Autodesk Fusion 360 part; units mm, degrees
(part 3 of 3)
sketch "Sketch2 (22)" plane through (0, 0, 0) normal (0, 0, 1) x (1, 0, 0) in component "04_RobotArm (2)"
  line L0 (-45, 50, 120) -> (11, 50, 120)
  line L1 (11, 50, 120) -> (11, 106, 120)
  line L2 (11, 106, 120) -> (-45, 106, 120)
  line L3 (-45, 106, 120) -> (-45, 50, 120)
extrude "Extrude2'''''''''''''''''''''" add sketch "Sketch2 (22)" along normal blind 76 separate body contours L0 L1 L2 L3 in plane through (0, 0, 120) normal (0, 0, 1) makes body 220 in component "04_RobotArm (2)"
sketch "Sketch3 (20)" plane through (0, 0, 0) normal (0, 0, 1) x (1, 0, 0) in component "04_RobotArm (2)"
  line L0 (-20, -20, 190) -> (20, -20, 190)
  line L1 (20, -20, 190) -> (20, 20, 190)
  line L2 (20, 20, 190) -> (-20, 20, 190)
  line L3 (-20, 20, 190) -> (-20, -20, 190)
extrude "Extrude3'''''''''''''''''''" add sketch "Sketch3 (20)" along normal blind 400 separate body contours L0 L1 L2 L3 in plane through (0, 0, 190) normal (0, 0, 1) makes body 221 in component "04_RobotArm (2)"
sketch "Sketch4 (20)" plane through (0, 0, 0) normal (0, 0, 1) x (1, 0, 0) in component "04_RobotArm (2)"
  line L0 (-25, -25, 250) -> (25, -25, 250)
  line L1 (25, -25, 250) -> (25, 25, 250)
  line L2 (25, 25, 250) -> (-25, 25, 250)
  line L3 (-25, 25, 250) -> (-25, -25, 250)
extrude "Extrude4'''''''''''''''''''" add sketch "Sketch4 (20)" along normal blind 5 separate body contours L0 L1 L2 L3 in plane through (0, 0, 250) normal (0, 0, 1) makes body 222 in component "04_RobotArm (2)"
sketch "Sketch5 (17)" plane through (0, 0, 0) normal (0, 0, 1) x (1, 0, 0) in component "04_RobotArm (2)"
  line L0 (-25, -25, 350) -> (25, -25, 350)
  line L1 (25, -25, 350) -> (25, 25, 350)
  line L2 (25, 25, 350) -> (-25, 25, 350)
  line L3 (-25, 25, 350) -> (-25, -25, 350)
extrude "Extrude5''''''''''''''''" add sketch "Sketch5 (17)" along normal blind 5 separate body contours L0 L1 L2 L3 in plane through (0, 0, 350) normal (0, 0, 1) makes body 223 in component "04_RobotArm (2)"
sketch "Sketch6 (17)" plane through (0, 0, 0) normal (0, 0, 1) x (1, 0, 0) in component "04_RobotArm (2)"
  line L0 (-25, -25, 450) -> (25, -25, 450)
  line L1 (25, -25, 450) -> (25, 25, 450)
  line L2 (25, 25, 450) -> (-25, 25, 450)
  line L3 (-25, 25, 450) -> (-25, -25, 450)
extrude "Extrude6''''''''''''''''" add sketch "Sketch6 (17)" along normal blind 5 separate body contours L0 L1 L2 L3 in plane through (0, 0, 450) normal (0, 0, 1) makes body 224 in component "04_RobotArm (2)"
sketch "Sketch7 (17)" plane through (0, 0, 0) normal (0, 0, 1) x (1, 0, 0) in component "04_RobotArm (2)"
  circle A0 through (60, 0, 590) (-30, 51.9615, 590) (-30, -51.9615, 590)
extrude "Extrude7''''''''''''''''" add sketch "Sketch7 (17)" along normal blind 40 separate body contours A0 in plane through (0, 0, 590) normal (0, 0, 1) makes body 225 in component "04_RobotArm (2)"
sketch "Sketch8 (17)" plane through (0, 0, 0) normal (0, 0, 1) x (1, 0, 0) in component "04_RobotArm (2)"
  line L0 (50, -30, 570) -> (106, -30, 570)
  line L1 (106, -30, 570) -> (106, 26, 570)
  line L2 (106, 26, 570) -> (50, 26, 570)
  line L3 (50, 26, 570) -> (50, -30, 570)
extrude "Extrude8''''''''''''''''" add sketch "Sketch8 (17)" along normal blind 76 separate body contours L0 L1 L2 L3 in plane through (0, 0, 570) normal (0, 0, 1) makes body 226 in component "04_RobotArm (2)"
sketch "Sketch9 (17)" plane through (0, 0, 0) normal (0, 0, 1) x (1, 0, 0) in component "04_RobotArm (2)"
  line L0 (-20, -20, 630) -> (20, -20, 630)
  line L1 (20, -20, 630) -> (20, 20, 630)
  line L2 (20, 20, 630) -> (-20, 20, 630)
  line L3 (-20, 20, 630) -> (-20, -20, 630)
extrude "Extrude9''''''''''''''''" add sketch "Sketch9 (17)" along normal blind 350 separate body contours L0 L1 L2 L3 in plane through (0, 0, 630) normal (0, 0, 1) makes body 227 in component "04_RobotArm (2)"
sketch "Sketch10 (17)" plane through (0, 0, 0) normal (0, 0, 1) x (1, 0, 0) in component "04_RobotArm (2)"
  circle A0 through (50, 0, 980) (-25, 43.3013, 980) (-25, -43.3013, 980)
extrude "Extrude10''''''''''''''''" add sketch "Sketch10 (17)" along normal blind 30 separate body contours A0 in plane through (0, 0, 980) normal (0, 0, 1) makes body 228 in component "04_RobotArm (2)"
sketch "Sketch11 (9)" plane through (0, 0, 0) normal (0, 0, 1) x (1, 0, 0) in component "04_RobotArm (2)"
  line L0 (30, -20, 960) -> (70, -20, 960)
  line L1 (70, -20, 960) -> (70, 20, 960)
  line L2 (70, 20, 960) -> (30, 20, 960)
  line L3 (30, 20, 960) -> (30, -20, 960)
extrude "Extrude11''''''''" add sketch "Sketch11 (9)" along normal blind 50 separate body contours L0 L1 L2 L3 in plane through (0, 0, 960) normal (0, 0, 1) makes body 229 in component "04_RobotArm (2)"
sketch "Sketch12 (7)" plane through (0, 0, 0) normal (0, 0, 1) x (1, 0, 0) in component "04_RobotArm (2)"
  circle A0 through (-15, 30, 130) (-37.5, 42.9904, 130) (-37.5, 17.0096, 130)
extrude "Extrude12''''''" add sketch "Sketch12 (7)" along normal blind 15 separate body contours A0 in plane through (0, 0, 130) normal (0, 0, 1) makes body 230 in component "04_RobotArm (2)"
sketch "Sketch13 (7)" plane through (0, 0, 0) normal (0, 0, 1) x (1, 0, 0) in component "04_RobotArm (2)"
  circle A0 through (-15, 30, 570) (-37.5, 42.9904, 570) (-37.5, 17.0096, 570)
extrude "Extrude13''''''" add sketch "Sketch13 (7)" along normal blind 15 separate body contours A0 in plane through (0, 0, 570) normal (0, 0, 1) makes body 231 in component "04_RobotArm (2)"
sketch "Sketch14 (7)" plane through (0, 0, 0) normal (0, 0, 1) x (1, 0, 0) in component "04_RobotArm (2)"
  circle A0 through (-15, 30, 960) (-37.5, 42.9904, 960) (-37.5, 17.0096, 960)
extrude "Extrude14''''''" add sketch "Sketch14 (7)" along normal blind 15 separate body contours A0 in plane through (0, 0, 960) normal (0, 0, 1) makes body 232 in component "04_RobotArm (2)"
sketch "Sketch1 (23)" plane through (0, 0, 0) normal (0, 0, 1) x (1, 0, 0) in component "05_Gripper (2)"
  line L0 (-50, -30) -> (50, -30)
  line L1 (50, -30) -> (50, 30)
  line L2 (50, 30) -> (-50, 30)
  line L3 (-50, 30) -> (-50, -30)
extrude "Extrude1''''''''''''''''''''''" add sketch "Sketch1 (23)" along normal blind 60 separate body makes body 233 in component "05_Gripper (2)"
sketch "Sketch2 (23)" plane through (0, 0, 0) normal (0, 0, 1) x (1, 0, 0) in component "05_Gripper (2)"
  line L0 (-75, -30) -> (-50, -30)
  line L1 (-50, -30) -> (-50, 30)
  line L2 (-50, 30) -> (-75, 30)
  line L3 (-75, 30) -> (-75, -30)
extrude "Extrude2''''''''''''''''''''''" add sketch "Sketch2 (23)" along normal blind 50 separate body makes body 234 in component "05_Gripper (2)"
sketch "Sketch3 (21)" plane through (0, 0, 0) normal (0, 0, 1) x (1, 0, 0) in component "05_Gripper (2)"
  line L0 (50, -30) -> (75, -30)
  line L1 (75, -30) -> (75, 30)
  line L2 (75, 30) -> (50, 30)
  line L3 (50, 30) -> (50, -30)
extrude "Extrude3''''''''''''''''''''" add sketch "Sketch3 (21)" along normal blind 50 separate body makes body 235 in component "05_Gripper (2)"
sketch "Sketch4 (21)" plane through (0, 0, 0) normal (0, 0, 1) x (1, 0, 0) in component "05_Gripper (2)"
  line L0 (-50, -25, 10) -> (50, -25, 10)
  line L1 (50, -25, 10) -> (50, -21, 10)
  line L2 (50, -21, 10) -> (-50, -21, 10)
  line L3 (-50, -21, 10) -> (-50, -25, 10)
extrude "Extrude4''''''''''''''''''''" add sketch "Sketch4 (21)" along normal blind 30 separate body contours L0 L1 L2 L3 in plane through (0, 0, 10) normal (0, 0, 1) makes body 236 in component "05_Gripper (2)"
sketch "Sketch5 (18)" plane through (0, 0, 0) normal (0, 0, 1) x (1, 0, 0) in component "05_Gripper (2)"
  line L0 (-50, 25, 10) -> (50, 25, 10)
  line L1 (50, 25, 10) -> (50, 29, 10)
  line L2 (50, 29, 10) -> (-50, 29, 10)
  line L3 (-50, 29, 10) -> (-50, 25, 10)
extrude "Extrude5'''''''''''''''''" add sketch "Sketch5 (18)" along normal blind 30 separate body contours L0 L1 L2 L3 in plane through (0, 0, 10) normal (0, 0, 1) makes body 237 in component "05_Gripper (2)"
sketch "Sketch6 (18)" plane through (0, 0, 0) normal (0, 0, 1) x (1, 0, 0) in component "05_Gripper (2)"
  circle A0 through (25, 0, 60) (-12.5, 21.6506, 60) (-12.5, -21.6506, 60)
extrude "Extrude6'''''''''''''''''" add sketch "Sketch6 (18)" along normal blind 80 separate body contours A0 in plane through (0, 0, 60) normal (0, 0, 1) makes body 238 in component "05_Gripper (2)"
sketch "Sketch7 (18)" plane through (0, 0, 0) normal (0, 0, 1) x (1, 0, 0) in component "05_Gripper (2)"
  circle A0 through (-16, 0, 140) (-22, 3.4641, 140) (-22, -3.4641, 140)
extrude "Extrude7'''''''''''''''''" add sketch "Sketch7 (18)" along normal blind 30 separate body contours A0 in plane through (0, 0, 140) normal (0, 0, 1) makes body 239 in component "05_Gripper (2)"
sketch "Sketch8 (18)" plane through (0, 0, 0) normal (0, 0, 1) x (1, 0, 0) in component "05_Gripper (2)"
  circle A0 through (24, 0, 140) (18, 3.4641, 140) (18, -3.4641, 140)
extrude "Extrude8'''''''''''''''''" add sketch "Sketch8 (18)" along normal blind 30 separate body contours A0 in plane through (0, 0, 140) normal (0, 0, 1) makes body 240 in component "05_Gripper (2)"
sketch "Sketch9 (18)" plane through (0, 0, 0) normal (0, 0, 1) x (1, 0, 0) in component "05_Gripper (2)"
  circle A0 through (30, 0, -20) (-15, 25.9808, -20) (-15, -25.9808, -20)
extrude "Extrude9'''''''''''''''''" add sketch "Sketch9 (18)" along normal blind 20 separate body contours A0 in plane through (0, 0, -20) normal (0, 0, 1) makes body 241 in component "05_Gripper (2)"
sketch "Sketch10 (18)" plane through (0, 0, 0) normal (0, 0, 1) x (1, 0, 0) in component "05_Gripper (2)"
  line L0 (-10, -5, -5) -> (10, -5, -5)
  line L1 (10, -5, -5) -> (10, 5, -5)
  line L2 (10, 5, -5) -> (-10, 5, -5)
  line L3 (-10, 5, -5) -> (-10, -5, -5)
extrude "Extrude10'''''''''''''''''" add sketch "Sketch10 (18)" along normal blind 3 separate body contours L0 L1 L2 L3 in plane through (0, 0, -5) normal (0, 0, 1) makes body 242 in component "05_Gripper (2)"
sketch "Sketch11 (10)" plane through (0, 0, 0) normal (0, 0, 1) x (1, 0, 0) in component "05_Gripper (2)"
  line L0 (-35, 35, 20) -> (35, 35, 20)
  line L1 (35, 35, 20) -> (35, 65, 20)
  line L2 (35, 65, 20) -> (-35, 65, 20)
  line L3 (-35, 65, 20) -> (-35, 35, 20)
extrude "Extrude11'''''''''" add sketch "Sketch11 (10)" along normal blind 40 separate body contours L0 L1 L2 L3 in plane through (0, 0, 20) normal (0, 0, 1) makes body 243 in component "05_Gripper (2)"
sketch "Sketch1 (24)" plane through (0, 0, 0) normal (0, 0, 1) x (1, 0, 0) in component "06_SortingBins (2)"
  line L0 (396.8309, 88.1111) -> (636.8309, 88.1111)
  line L1 (636.8309, 88.1111) -> (636.8309, 288.1111)
  line L2 (636.8309, 288.1111) -> (396.8309, 288.1111)
  line L3 (396.8309, 288.1111) -> (396.8309, 88.1111)
extrude "Extrude1'''''''''''''''''''''''" add sketch "Sketch1 (24)" along normal blind 250 separate body makes body 244 in component "06_SortingBins (2)"
sketch "Sketch2 (24)" plane through (0, 0, 0) normal (0, 0, 1) x (1, 0, 0) in component "06_SortingBins (2)"
  line L0 (456.8309, 83.1111, 80) -> (576.8309, 83.1111, 80)
  line L1 (576.8309, 83.1111, 80) -> (576.8309, 86.1111, 80)
  line L2 (576.8309, 86.1111, 80) -> (456.8309, 86.1111, 80)
  line L3 (456.8309, 86.1111, 80) -> (456.8309, 83.1111, 80)
extrude "Extrude2'''''''''''''''''''''''" add sketch "Sketch2 (24)" along normal blind 60 separate body contours L0 L1 L2 L3 in plane through (0, 0, 80) normal (0, 0, 1) makes body 245 in component "06_SortingBins (2)"
sketch "Sketch3 (22)" plane through (0, 0, 0) normal (0, 0, 1) x (1, 0, 0) in component "06_SortingBins (2)"
  line L0 (396.8309, 88.1111, -15) -> (636.8309, 88.1111, -15)
  line L1 (636.8309, 88.1111, -15) -> (636.8309, 288.1111, -15)
  line L2 (636.8309, 288.1111, -15) -> (396.8309, 288.1111, -15)
  line L3 (396.8309, 288.1111, -15) -> (396.8309, 88.1111, -15)
extrude "Extrude3'''''''''''''''''''''" add sketch "Sketch3 (22)" along normal blind 15 separate body contours L0 L1 L2 L3 in plane through (0, 0, -15) normal (0, 0, 1) makes body 246 in component "06_SortingBins (2)"
sketch "Sketch4 (22)" plane through (0, 0, 0) normal (0, 0, 1) x (1, 0, 0) in component "06_SortingBins (2)"
  line L0 (280.0555, 277.4329) -> (520.0555, 277.4329)
  line L1 (520.0555, 277.4329) -> (520.0555, 477.4329)
  line L2 (520.0555, 477.4329) -> (280.0555, 477.4329)
  line L3 (280.0555, 477.4329) -> (280.0555, 277.4329)
extrude "Extrude4'''''''''''''''''''''" add sketch "Sketch4 (22)" along normal blind 250 separate body makes body 247 in component "06_SortingBins (2)"
sketch "Sketch5 (19)" plane through (0, 0, 0) normal (0, 0, 1) x (1, 0, 0) in component "06_SortingBins (2)"
  line L0 (340.0555, 272.4329, 80) -> (460.0555, 272.4329, 80)
  line L1 (460.0555, 272.4329, 80) -> (460.0555, 275.4329, 80)
  line L2 (460.0555, 275.4329, 80) -> (340.0555, 275.4329, 80)
  line L3 (340.0555, 275.4329, 80) -> (340.0555, 272.4329, 80)
extrude "Extrude5''''''''''''''''''" add sketch "Sketch5 (19)" along normal blind 60 separate body contours L0 L1 L2 L3 in plane through (0, 0, 80) normal (0, 0, 1) makes body 248 in component "06_SortingBins (2)"
sketch "Sketch6 (19)" plane through (0, 0, 0) normal (0, 0, 1) x (1, 0, 0) in component "06_SortingBins (2)"
  line L0 (280.0555, 277.4329, -15) -> (520.0555, 277.4329, -15)
  line L1 (520.0555, 277.4329, -15) -> (520.0555, 477.4329, -15)
  line L2 (520.0555, 477.4329, -15) -> (280.0555, 477.4329, -15)
  line L3 (280.0555, 477.4329, -15) -> (280.0555, 277.4329, -15)
extrude "Extrude6''''''''''''''''''" add sketch "Sketch6 (19)" along normal blind 15 separate body contours L0 L1 L2 L3 in plane through (0, 0, -15) normal (0, 0, 1) makes body 249 in component "06_SortingBins (2)"
sketch "Sketch7 (19)" plane through (0, 0, 0) normal (0, 0, 1) x (1, 0, 0) in component "06_SortingBins (2)"
  line L0 (97.8439, 405.0189) -> (337.8439, 405.0189)
  line L1 (337.8439, 405.0189) -> (337.8439, 605.0189)
  line L2 (337.8439, 605.0189) -> (97.8439, 605.0189)
  line L3 (97.8439, 605.0189) -> (97.8439, 405.0189)
extrude "Extrude7''''''''''''''''''" add sketch "Sketch7 (19)" along normal blind 250 separate body makes body 250 in component "06_SortingBins (2)"
sketch "Sketch8 (19)" plane through (0, 0, 0) normal (0, 0, 1) x (1, 0, 0) in component "06_SortingBins (2)"
  line L0 (157.8439, 400.0189, 80) -> (277.8439, 400.0189, 80)
  line L1 (277.8439, 400.0189, 80) -> (277.8439, 403.0189, 80)
  line L2 (277.8439, 403.0189, 80) -> (157.8439, 403.0189, 80)
  line L3 (157.8439, 403.0189, 80) -> (157.8439, 400.0189, 80)
extrude "Extrude8''''''''''''''''''" add sketch "Sketch8 (19)" along normal blind 60 separate body contours L0 L1 L2 L3 in plane through (0, 0, 80) normal (0, 0, 1) makes body 251 in component "06_SortingBins (2)"
sketch "Sketch9 (19)" plane through (0, 0, 0) normal (0, 0, 1) x (1, 0, 0) in component "06_SortingBins (2)"
  line L0 (97.8439, 405.0189, -15) -> (337.8439, 405.0189, -15)
  line L1 (337.8439, 405.0189, -15) -> (337.8439, 605.0189, -15)
  line L2 (337.8439, 605.0189, -15) -> (97.8439, 605.0189, -15)
  line L3 (97.8439, 605.0189, -15) -> (97.8439, 405.0189, -15)
extrude "Extrude9''''''''''''''''''" add sketch "Sketch9 (19)" along normal blind 15 separate body contours L0 L1 L2 L3 in plane through (0, 0, -15) normal (0, 0, 1) makes body 252 in component "06_SortingBins (2)"
sketch "Sketch10 (19)" plane through (0, 0, 0) normal (0, 0, 1) x (1, 0, 0) in component "06_SortingBins (2)"
  line L0 (-120, 450) -> (120, 450)
  line L1 (120, 450) -> (120, 650)
  line L2 (120, 650) -> (-120, 650)
  line L3 (-120, 650) -> (-120, 450)
extrude "Extrude10''''''''''''''''''" add sketch "Sketch10 (19)" along normal blind 250 separate body makes body 253 in component "06_SortingBins (2)"
sketch "Sketch11 (11)" plane through (0, 0, 0) normal (0, 0, 1) x (1, 0, 0) in component "06_SortingBins (2)"
  line L0 (-60, 445, 80) -> (60, 445, 80)
  line L1 (60, 445, 80) -> (60, 448, 80)
  line L2 (60, 448, 80) -> (-60, 448, 80)
  line L3 (-60, 448, 80) -> (-60, 445, 80)
extrude "Extrude11''''''''''" add sketch "Sketch11 (11)" along normal blind 60 separate body contours L0 L1 L2 L3 in plane through (0, 0, 80) normal (0, 0, 1) makes body 254 in component "06_SortingBins (2)"
sketch "Sketch12 (8)" plane through (0, 0, 0) normal (0, 0, 1) x (1, 0, 0) in component "06_SortingBins (2)"
  line L0 (-120, 450, -15) -> (120, 450, -15)
  line L1 (120, 450, -15) -> (120, 650, -15)
  line L2 (120, 650, -15) -> (-120, 650, -15)
  line L3 (-120, 650, -15) -> (-120, 450, -15)
extrude "Extrude12'''''''" add sketch "Sketch12 (8)" along normal blind 15 separate body contours L0 L1 L2 L3 in plane through (0, 0, -15) normal (0, 0, 1) makes body 255 in component "06_SortingBins (2)"
sketch "Sketch13 (8)" plane through (0, 0, 0) normal (0, 0, 1) x (1, 0, 0) in component "06_SortingBins (2)"
  line L0 (-337.8439, 405.0189) -> (-97.8439, 405.0189)
  line L1 (-97.8439, 405.0189) -> (-97.8439, 605.0189)
  line L2 (-97.8439, 605.0189) -> (-337.8439, 605.0189)
  line L3 (-337.8439, 605.0189) -> (-337.8439, 405.0189)
extrude "Extrude13'''''''" add sketch "Sketch13 (8)" along normal blind 250 separate body makes body 256 in component "06_SortingBins (2)"
sketch "Sketch14 (8)" plane through (0, 0, 0) normal (0, 0, 1) x (1, 0, 0) in component "06_SortingBins (2)"
  line L0 (-277.8439, 400.0189, 80) -> (-157.8439, 400.0189, 80)
  line L1 (-157.8439, 400.0189, 80) -> (-157.8439, 403.0189, 80)
  line L2 (-157.8439, 403.0189, 80) -> (-277.8439, 403.0189, 80)
  line L3 (-277.8439, 403.0189, 80) -> (-277.8439, 400.0189, 80)
extrude "Extrude14'''''''" add sketch "Sketch14 (8)" along normal blind 60 separate body contours L0 L1 L2 L3 in plane through (0, 0, 80) normal (0, 0, 1) makes body 257 in component "06_SortingBins (2)"
sketch "Sketch15 (5)" plane through (0, 0, 0) normal (0, 0, 1) x (1, 0, 0) in component "06_SortingBins (2)"
  line L0 (-337.8439, 405.0189, -15) -> (-97.8439, 405.0189, -15)
  line L1 (-97.8439, 405.0189, -15) -> (-97.8439, 605.0189, -15)
  line L2 (-97.8439, 605.0189, -15) -> (-337.8439, 605.0189, -15)
  line L3 (-337.8439, 605.0189, -15) -> (-337.8439, 405.0189, -15)
extrude "Extrude15''''" add sketch "Sketch15 (5)" along normal blind 15 separate body contours L0 L1 L2 L3 in plane through (0, 0, -15) normal (0, 0, 1) makes body 258 in component "06_SortingBins (2)"
sketch "Sketch16 (3)" plane through (0, 0, 0) normal (0, 0, 1) x (1, 0, 0) in component "06_SortingBins (2)"
  line L0 (-520.0555, 277.4329) -> (-280.0555, 277.4329)
  line L1 (-280.0555, 277.4329) -> (-280.0555, 477.4329)
  line L2 (-280.0555, 477.4329) -> (-520.0555, 477.4329)
  line L3 (-520.0555, 477.4329) -> (-520.0555, 277.4329)
extrude "Extrude16''" add sketch "Sketch16 (3)" along normal blind 250 separate body makes body 259 in component "06_SortingBins (2)"
sketch "Sketch17 (3)" plane through (0, 0, 0) normal (0, 0, 1) x (1, 0, 0) in component "06_SortingBins (2)"
  line L0 (-460.0555, 272.4329, 80) -> (-340.0555, 272.4329, 80)
  line L1 (-340.0555, 272.4329, 80) -> (-340.0555, 275.4329, 80)
  line L2 (-340.0555, 275.4329, 80) -> (-460.0555, 275.4329, 80)
  line L3 (-460.0555, 275.4329, 80) -> (-460.0555, 272.4329, 80)
extrude "Extrude17''" add sketch "Sketch17 (3)" along normal blind 60 separate body contours L0 L1 L2 L3 in plane through (0, 0, 80) normal (0, 0, 1) makes body 260 in component "06_SortingBins (2)"
sketch "Sketch18 (3)" plane through (0, 0, 0) normal (0, 0, 1) x (1, 0, 0) in component "06_SortingBins (2)"
  line L0 (-520.0555, 277.4329, -15) -> (-280.0555, 277.4329, -15)
  line L1 (-280.0555, 277.4329, -15) -> (-280.0555, 477.4329, -15)
  line L2 (-280.0555, 477.4329, -15) -> (-520.0555, 477.4329, -15)
  line L3 (-520.0555, 477.4329, -15) -> (-520.0555, 277.4329, -15)
extrude "Extrude18''" add sketch "Sketch18 (3)" along normal blind 15 separate body contours L0 L1 L2 L3 in plane through (0, 0, -15) normal (0, 0, 1) makes body 261 in component "06_SortingBins (2)"
sketch "Sketch19 (3)" plane through (0, 0, 0) normal (0, 0, 1) x (1, 0, 0) in component "06_SortingBins (2)"
  line L0 (-636.8309, 88.1111) -> (-396.8309, 88.1111)
  line L1 (-396.8309, 88.1111) -> (-396.8309, 288.1111)
  line L2 (-396.8309, 288.1111) -> (-636.8309, 288.1111)
  line L3 (-636.8309, 288.1111) -> (-636.8309, 88.1111)
extrude "Extrude19''" add sketch "Sketch19 (3)" along normal blind 250 separate body makes body 262 in component "06_SortingBins (2)"
sketch "Sketch20 (3)" plane through (0, 0, 0) normal (0, 0, 1) x (1, 0, 0) in component "06_SortingBins (2)"
  line L0 (-576.8309, 83.1111, 80) -> (-456.8309, 83.1111, 80)
  line L1 (-456.8309, 83.1111, 80) -> (-456.8309, 86.1111, 80)
  line L2 (-456.8309, 86.1111, 80) -> (-576.8309, 86.1111, 80)
  line L3 (-576.8309, 86.1111, 80) -> (-576.8309, 83.1111, 80)
extrude "Extrude20''" add sketch "Sketch20 (3)" along normal blind 60 separate body contours L0 L1 L2 L3 in plane through (0, 0, 80) normal (0, 0, 1) makes body 263 in component "06_SortingBins (2)"
sketch "Sketch21 (3)" plane through (0, 0, 0) normal (0, 0, 1) x (1, 0, 0) in component "06_SortingBins (2)"
  line L0 (-636.8309, 88.1111, -15) -> (-396.8309, 88.1111, -15)
  line L1 (-396.8309, 88.1111, -15) -> (-396.8309, 288.1111, -15)
  line L2 (-396.8309, 288.1111, -15) -> (-636.8309, 288.1111, -15)
  line L3 (-636.8309, 288.1111, -15) -> (-636.8309, 88.1111, -15)
extrude "Extrude21''" add sketch "Sketch21 (3)" along normal blind 15 separate body contours L0 L1 L2 L3 in plane through (0, 0, -15) normal (0, 0, 1) makes body 264 in component "06_SortingBins (2)"
sketch "Sketch1 (25)" plane through (0, 0, 0) normal (0, 0, 1) x (1, 0, 0) in component "07_ComputeCabinet (2)"
  line L0 (0, 0) -> (500, 0)
  line L1 (500, 0) -> (500, 300)
  line L2 (500, 300) -> (0, 300)
  line L3 (0, 300) -> (0, 0)
extrude "Extrude1''''''''''''''''''''''''" add sketch "Sketch1 (25)" along normal blind 700 separate body makes body 265 in component "07_ComputeCabinet (2)"
sketch "Sketch2 (25)" plane through (0, 0, 0) normal (0, 0, 1) x (1, 0, 0) in component "07_ComputeCabinet (2)"
  line L0 (0, -5, 50) -> (500, -5, 50)
  line L1 (500, -5, 50) -> (500, 0, 50)
  line L2 (500, 0, 50) -> (0, 0, 50)
  line L3 (0, 0, 50) -> (0, -5, 50)
extrude "Extrude2''''''''''''''''''''''''" add sketch "Sketch2 (25)" along normal blind 600 separate body contours L0 L1 L2 L3 in plane through (0, 0, 50) normal (0, 0, 1) makes body 266 in component "07_ComputeCabinet (2)"
sketch "Sketch3 (23)" plane through (0, 0, 0) normal (0, 0, 1) x (1, 0, 0) in component "07_ComputeCabinet (2)"
  line L0 (30, 50, 120) -> (470, 50, 120)
  line L1 (470, 50, 120) -> (470, 54, 120)
  line L2 (470, 54, 120) -> (30, 54, 120)
  line L3 (30, 54, 120) -> (30, 50, 120)
extrude "Extrude3''''''''''''''''''''''" add sketch "Sketch3 (23)" along normal blind 15 separate body contours L0 L1 L2 L3 in plane through (0, 0, 120) normal (0, 0, 1) makes body 267 in component "07_ComputeCabinet (2)"
sketch "Sketch4 (23)" plane through (0, 0, 0) normal (0, 0, 1) x (1, 0, 0) in component "07_ComputeCabinet (2)"
  line L0 (30, 50, 300) -> (470, 50, 300)
  line L1 (470, 50, 300) -> (470, 54, 300)
  line L2 (470, 54, 300) -> (30, 54, 300)
  line L3 (30, 54, 300) -> (30, 50, 300)
extrude "Extrude4''''''''''''''''''''''" add sketch "Sketch4 (23)" along normal blind 15 separate body contours L0 L1 L2 L3 in plane through (0, 0, 300) normal (0, 0, 1) makes body 268 in component "07_ComputeCabinet (2)"
sketch "Sketch5 (20)" plane through (0, 0, 0) normal (0, 0, 1) x (1, 0, 0) in component "07_ComputeCabinet (2)"
  line L0 (30, 50, 500) -> (470, 50, 500)
  line L1 (470, 50, 500) -> (470, 54, 500)
  line L2 (470, 54, 500) -> (30, 54, 500)
  line L3 (30, 54, 500) -> (30, 50, 500)
extrude "Extrude5'''''''''''''''''''" add sketch "Sketch5 (20)" along normal blind 15 separate body contours L0 L1 L2 L3 in plane through (0, 0, 500) normal (0, 0, 1) makes body 269 in component "07_ComputeCabinet (2)"
sketch "Sketch6 (20)" plane through (0, 0, 0) normal (0, 0, 1) x (1, 0, 0) in component "07_ComputeCabinet (2)"
  line L0 (40, 60, 140) -> (140, 60, 140)
  line L1 (140, 60, 140) -> (140, 140, 140)
  line L2 (140, 140, 140) -> (40, 140, 140)
  line L3 (40, 140, 140) -> (40, 60, 140)
extrude "Extrude6'''''''''''''''''''" add sketch "Sketch6 (20)" along normal blind 60 separate body contours L0 L1 L2 L3 in plane through (0, 0, 140) normal (0, 0, 1) makes body 270 in component "07_ComputeCabinet (2)"
sketch "Sketch7 (20)" plane through (0, 0, 0) normal (0, 0, 1) x (1, 0, 0) in component "07_ComputeCabinet (2)"
  circle A0 through (120, 100, 200) (75, 125.9808, 200) (75, 74.0192, 200)
extrude "Extrude7'''''''''''''''''''" add sketch "Sketch7 (20)" along normal blind 10 separate body contours A0 in plane through (0, 0, 200) normal (0, 0, 1) makes body 271 in component "07_ComputeCabinet (2)"
sketch "Sketch8 (20)" plane through (0, 0, 0) normal (0, 0, 1) x (1, 0, 0) in component "07_ComputeCabinet (2)"
  line L0 (180, 60, 140) -> (240, 60, 140)
  line L1 (240, 60, 140) -> (240, 100, 140)
  line L2 (240, 100, 140) -> (180, 100, 140)
  line L3 (180, 100, 140) -> (180, 60, 140)
extrude "Extrude8'''''''''''''''''''" add sketch "Sketch8 (20)" along normal blind 10 separate body contours L0 L1 L2 L3 in plane through (0, 0, 140) normal (0, 0, 1) makes body 272 in component "07_ComputeCabinet (2)"
sketch "Sketch9 (20)" plane through (0, 0, 0) normal (0, 0, 1) x (1, 0, 0) in component "07_ComputeCabinet (2)"
  line L0 (270, 60, 140) -> (350, 60, 140)
  line L1 (350, 60, 140) -> (350, 80, 140)
  line L2 (350, 80, 140) -> (270, 80, 140)
  line L3 (270, 80, 140) -> (270, 60, 140)
extrude "Extrude9'''''''''''''''''''" add sketch "Sketch9 (20)" along normal blind 4 separate body contours L0 L1 L2 L3 in plane through (0, 0, 140) normal (0, 0, 1) makes body 273 in component "07_ComputeCabinet (2)"
sketch "Sketch10 (20)" plane through (0, 0, 0) normal (0, 0, 1) x (1, 0, 0) in component "07_ComputeCabinet (2)"
  line L0 (40, 60, 320) -> (220, 60, 320)
  line L1 (220, 60, 320) -> (220, 160, 320)
  line L2 (220, 160, 320) -> (40, 160, 320)
  line L3 (40, 160, 320) -> (40, 60, 320)
extrude "Extrude10'''''''''''''''''''" add sketch "Sketch10 (20)" along normal blind 60 separate body contours L0 L1 L2 L3 in plane through (0, 0, 320) normal (0, 0, 1) makes body 274 in component "07_ComputeCabinet (2)"
sketch "Sketch11 (12)" plane through (0, 0, 0) normal (0, 0, 1) x (1, 0, 0) in component "07_ComputeCabinet (2)"
  line L0 (260, 60, 320) -> (440, 60, 320)
  line L1 (440, 60, 320) -> (440, 160, 320)
  line L2 (440, 160, 320) -> (260, 160, 320)
  line L3 (260, 160, 320) -> (260, 60, 320)
extrude "Extrude11'''''''''''" add sketch "Sketch11 (12)" along normal blind 60 separate body contours L0 L1 L2 L3 in plane through (0, 0, 320) normal (0, 0, 1) makes body 275 in component "07_ComputeCabinet (2)"
sketch "Sketch12 (9)" plane through (0, 0, 0) normal (0, 0, 1) x (1, 0, 0) in component "07_ComputeCabinet (2)"
  line L0 (40, 60, 520) -> (420, 60, 520)
  line L1 (420, 60, 520) -> (420, 200, 520)
  line L2 (420, 200, 520) -> (40, 200, 520)
  line L3 (40, 200, 520) -> (40, 60, 520)
extrude "Extrude12''''''''" add sketch "Sketch12 (9)" along normal blind 100 separate body contours L0 L1 L2 L3 in plane through (0, 0, 520) normal (0, 0, 1) makes body 276 in component "07_ComputeCabinet (2)"
sketch "Sketch13 (9)" plane through (0, 0, 0) normal (0, 0, 1) x (1, 0, 0) in component "07_ComputeCabinet (2)"
  circle A0 through (80, -3, 550) (35, 22.9808, 550) (35, -28.9808, 550)
extrude "Extrude13''''''''" add sketch "Sketch13 (9)" along normal blind 30 separate body contours A0 in plane through (0, 0, 550) normal (0, 0, 1) makes body 277 in component "07_ComputeCabinet (2)"
sketch "Sketch14 (9)" plane through (0, 0, 0) normal (0, 0, 1) x (1, 0, 0) in component "07_ComputeCabinet (2)"
  line L0 (360, 60, 140) -> (420, 60, 140)
  line L1 (420, 60, 140) -> (420, 100, 140)
  line L2 (420, 100, 140) -> (360, 100, 140)
  line L3 (360, 100, 140) -> (360, 60, 140)
extrude "Extrude14''''''''" add sketch "Sketch14 (9)" along normal blind 40 separate body contours L0 L1 L2 L3 in plane through (0, 0, 140) normal (0, 0, 1) makes body 278 in component "07_ComputeCabinet (2)"
sketch "Sketch15 (6)" plane through (0, 0, 0) normal (0, 0, 1) x (1, 0, 0) in component "07_ComputeCabinet (2)"
  line L0 (180, 60, 220) -> (220, 60, 220)
  line L1 (220, 60, 220) -> (220, 85, 220)
  line L2 (220, 85, 220) -> (180, 85, 220)
  line L3 (180, 85, 220) -> (180, 60, 220)
extrude "Extrude15'''''" add sketch "Sketch15 (6)" along normal blind 3 separate body contours L0 L1 L2 L3 in plane through (0, 0, 220) normal (0, 0, 1) makes body 279 in component "07_ComputeCabinet (2)"
sketch "Sketch1 (26)" plane through (0, 0, 0) normal (0, 0, 1) x (1, 0, 0) in component "08_PneumaticSystem (2)"
  line L0 (0, 0) -> (300, 0)
  line L1 (300, 0) -> (300, 200)
  line L2 (300, 200) -> (0, 200)
  line L3 (0, 200) -> (0, 0)
extrude "Extrude1'''''''''''''''''''''''''" add sketch "Sketch1 (26)" along normal blind 350 separate body makes body 280 in component "08_PneumaticSystem (2)"
sketch "Sketch2 (26)" plane through (0, 0, 0) normal (0, 0, 1) x (1, 0, 0) in component "08_PneumaticSystem (2)"
  circle A0 through (230, 100, 350) (110, 169.282, 350) (110, 30.718, 350)
extrude "Extrude2'''''''''''''''''''''''''" add sketch "Sketch2 (26)" along normal blind 200 separate body contours A0 in plane through (0, 0, 350) normal (0, 0, 1) makes body 281 in component "08_PneumaticSystem (2)"
sketch "Sketch3 (24)" plane through (0, 0, 0) normal (0, 0, 1) x (1, 0, 0) in component "08_PneumaticSystem (2)"
  line L0 (0, 220, 150) -> (200, 220, 150)
  line L1 (200, 220, 150) -> (200, 300, 150)
  line L2 (200, 300, 150) -> (0, 300, 150)
  line L3 (0, 300, 150) -> (0, 220, 150)
extrude "Extrude3'''''''''''''''''''''''" add sketch "Sketch3 (24)" along normal blind 60 separate body contours L0 L1 L2 L3 in plane through (0, 0, 150) normal (0, 0, 1) makes body 282 in component "08_PneumaticSystem (2)"
sketch "Sketch4 (24)" plane through (0, 0, 0) normal (0, 0, 1) x (1, 0, 0) in component "08_PneumaticSystem (2)"
  line L0 (20, 220, 210) -> (60, 220, 210)
  line L1 (60, 220, 210) -> (60, 280, 210)
  line L2 (60, 280, 210) -> (20, 280, 210)
  line L3 (20, 280, 210) -> (20, 220, 210)
extrude "Extrude4'''''''''''''''''''''''" add sketch "Sketch4 (24)" along normal blind 40 separate body contours L0 L1 L2 L3 in plane through (0, 0, 210) normal (0, 0, 1) makes body 283 in component "08_PneumaticSystem (2)"
sketch "Sketch5 (21)" plane through (0, 0, 0) normal (0, 0, 1) x (1, 0, 0) in component "08_PneumaticSystem (2)"
  line L0 (80, 220, 210) -> (120, 220, 210)
  line L1 (120, 220, 210) -> (120, 280, 210)
  line L2 (120, 280, 210) -> (80, 280, 210)
  line L3 (80, 280, 210) -> (80, 220, 210)
extrude "Extrude5''''''''''''''''''''" add sketch "Sketch5 (21)" along normal blind 40 separate body contours L0 L1 L2 L3 in plane through (0, 0, 210) normal (0, 0, 1) makes body 284 in component "08_PneumaticSystem (2)"
sketch "Sketch6 (21)" plane through (0, 0, 0) normal (0, 0, 1) x (1, 0, 0) in component "08_PneumaticSystem (2)"
  line L0 (140, 220, 210) -> (180, 220, 210)
  line L1 (180, 220, 210) -> (180, 280, 210)
  line L2 (180, 280, 210) -> (140, 280, 210)
  line L3 (140, 280, 210) -> (140, 220, 210)
extrude "Extrude6''''''''''''''''''''" add sketch "Sketch6 (21)" along normal blind 40 separate body contours L0 L1 L2 L3 in plane through (0, 0, 210) normal (0, 0, 1) makes body 285 in component "08_PneumaticSystem (2)"
sketch "Sketch7 (21)" plane through (0, 0, 0) normal (0, 0, 1) x (1, 0, 0) in component "08_PneumaticSystem (2)"
  circle A0 through (195, 260, 150) (157.5, 281.6506, 150) (157.5, 238.3494, 150)
extrude "Extrude7''''''''''''''''''''" add sketch "Sketch7 (21)" along normal blind 70 separate body contours A0 in plane through (0, 0, 150) normal (0, 0, 1) makes body 286 in component "08_PneumaticSystem (2)"
sketch "Sketch8 (21)" plane through (0, 0, 0) normal (0, 0, 1) x (1, 0, 0) in component "08_PneumaticSystem (2)"
  circle A0 through (50, 260, 150) (20, 277.3205, 150) (20, 242.6795, 150)
extrude "Extrude8''''''''''''''''''''" add sketch "Sketch8 (21)" along normal blind 60 separate body contours A0 in plane through (0, 0, 150) normal (0, 0, 1) makes body 287 in component "08_PneumaticSystem (2)"
sketch "Sketch9 (21)" plane through (0, 0, 0) normal (0, 0, 1) x (1, 0, 0) in component "08_PneumaticSystem (2)"
  line L0 (200, 100, 200) -> (208, 100, 200)
  line L1 (208, 100, 200) -> (208, 250, 200)
  line L2 (208, 250, 200) -> (200, 250, 200)
  line L3 (200, 250, 200) -> (200, 100, 200)
extrude "Extrude9''''''''''''''''''''" add sketch "Sketch9 (21)" along normal blind 8 separate body contours L0 L1 L2 L3 in plane through (0, 0, 200) normal (0, 0, 1) makes body 288 in component "08_PneumaticSystem (2)"
sketch "Sketch10 (21)" plane through (0, 0, 0) normal (0, 0, 1) x (1, 0, 0) in component "08_PneumaticSystem (2)"
  line L0 (230, 100, 200) -> (238, 100, 200)
  line L1 (238, 100, 200) -> (238, 250, 200)
  line L2 (238, 250, 200) -> (230, 250, 200)
  line L3 (230, 250, 200) -> (230, 100, 200)
extrude "Extrude10''''''''''''''''''''" add sketch "Sketch10 (21)" along normal blind 8 separate body contours L0 L1 L2 L3 in plane through (0, 0, 200) normal (0, 0, 1) makes body 289 in component "08_PneumaticSystem (2)"
sketch "Sketch1 (27)" plane through (0, 0, 0) normal (0, 0, 1) x (1, 0, 0) in component "09_TriggerSensor (2)"
  line L0 (780, -50, 100) -> (800, -50, 100)
  line L1 (800, -50, 100) -> (800, -20, 100)
  line L2 (800, -20, 100) -> (780, -20, 100)
  line L3 (780, -20, 100) -> (780, -50, 100)
component "01_ConveyorBelt" placed x (1, 0, 0) y (0, 1, 0) z (0, 0, 1) at (0, 0, 0)
component "02_VisionStation" placed x (1, 0, 0) y (0, 1, 0) z (0, 0, 1) at (0, 0, 0)
component "03_RobotBase" placed x (1, 0, 0) y (0, 1, 0) z (0, 0, 1) at (1500, 600, 0)
component "04_RobotArm" placed x (1, 0, 0) y (0, 1, 0) z (0, 0, 1) at (1500, 600, 100)
component "05_Gripper" placed x (1, 0, 0) y (0, 1, 0) z (0, 0, 1) at (1500, 600, 1060)
component "06_SortingBins" placed x (1, 0, 0) y (0, 1, 0) z (0, 0, 1) at (1500, 600, 0)
component "07_ComputeCabinet" placed x (1, 0, 0) y (0, 1, 0) z (0, 0, 1) at (-600, 0, 0)
component "08_PneumaticSystem" placed x (1, 0, 0) y (0, 1, 0) z (0, 0, 1) at (-600, 400, 0)
component "09_TriggerSensor" placed x (1, 0, 0) y (0, 1, 0) z (0, 0, 1) at (0, 0, 0)
component "01_ConveyorBelt (1)" placed x (1, 0, 0) y (0, 1, 0) z (0, 0, 1) at (0, 0, 0)
component "02_VisionStation (1)" placed x (1, 0, 0) y (0, 1, 0) z (0, 0, 1) at (0, 0, 0)
component "03_RobotBase (1)" placed x (1, 0, 0) y (0, 1, 0) z (0, 0, 1) at (1500, 600, 0)
component "04_RobotArm (1)" placed x (1, 0, 0) y (0, 1, 0) z (0, 0, 1) at (1500, 600, 100)
component "05_Gripper (1)" placed x (1, 0, 0) y (0, 1, 0) z (0, 0, 1) at (1500, 600, 1080)
component "06_SortingBins (1)" placed x (1, 0, 0) y (0, 1, 0) z (0, 0, 1) at (1500, 600, 0)
component "07_ComputeCabinet (1)" placed x (1, 0, 0) y (0, 1, 0) z (0, 0, 1) at (-600, 0, 0)
component "08_PneumaticSystem (1)" placed x (1, 0, 0) y (0, 1, 0) z (0, 0, 1) at (-600, 400, 0)
component "09_TriggerSensor (1)" placed x (1, 0, 0) y (0, 1, 0) z (0, 0, 1) at (0, 0, 0)
component "01_ConveyorBelt (2)" placed x (1, 0, 0) y (0, 1, 0) z (0, 0, 1) at (0, 0, 0)
component "02_VisionStation (2)" placed x (1, 0, 0) y (0, 1, 0) z (0, 0, 1) at (0, 0, 0)
component "03_RobotBase (2)" placed x (1, 0, 0) y (0, 1, 0) z (0, 0, 1) at (1500, 600, 0)
component "04_RobotArm (2)" placed x (1, 0, 0) y (0, 1, 0) z (0, 0, 1) at (1500, 600, 100)
component "05_Gripper (2)" placed x (1, 0, 0) y (0, 1, 0) z (0, 0, 1) at (1500, 600, 1080)
component "06_SortingBins (2)" placed x (1, 0, 0) y (0, 1, 0) z (0, 0, 1) at (1500, 600, 0)
component "07_ComputeCabinet (2)" placed x (1, 0, 0) y (0, 1, 0) z (0, 0, 1) at (-600, 0, 0)
component "08_PneumaticSystem (2)" placed x (1, 0, 0) y (0, 1, 0) z (0, 0, 1) at (-600, 400, 0)
component "09_TriggerSensor (2)" placed x (1, 0, 0) y (0, 1, 0) z (0, 0, 1) at (0, 0, 0)
component "01_ConveyorBelt" placed x (1, 0, 0) y (0, 1, 0) z (0, 0, 1) at (0, 0, 0) in component "07_ComputeCabinet"
named bodies: "Leg", "Leg (1)", "Leg (2)", "Leg (3)", "Rail_Front", "Rail_Back", "BeltSurface", "Roller", "Roller (1)", "BeltMotor", "ArchPost_L", "ArchPost_R", "ArchBar", "CamMount", "RGBCamera", "CamLens", "RealSense_D455", "DepthLens", "DepthLens (1)", "LEDRing", "AnchorPlate", "BaseCylinder", "Turntable", "TurntableMotor", "ShoulderJoint", "ShoulderMotor", "UpperArm", "Rib", "Rib (1)", "Rib (2)", "ElbowJoint", "ElbowMotor", "Forearm", "WristJoint", "WristMotor", "Encoder", "Encoder (1)", "Encoder (2)", "GripperBody", "Jaw_Left", "Jaw_Right", "JawRail", "JawRail (1)", "PneumCylinder", "HosePort", "HosePort (1)", "VacuumPad", "ForceSensor", "SolenoidValve", "Bin_PET", "Label_PET", "LoadCell_PET", "Bin_HDPE", "Label_HDPE", "LoadCell_HDPE", "Bin_PVC", "Label_PVC", "LoadCell_PVC", "Bin_LDPE", "Label_LDPE", "LoadCell_LDPE", "Bin_PP", "Label_PP", "LoadCell_PP", "Bin_PS", "Label_PS", "LoadCell_PS", "Bin_OTHER", "Label_OTHER", "LoadCell_OTHER", "Cabinet", "Door", "DINRail", "DINRail (1)", "DINRail (2)", "Jetson_AGX_Orin", "JetsonFan", "STM32H7", "NVMe_SSD", "PSU", "PSU (1)", "UPS_Battery", "EStop", "SafetyRelay", "PCA9685", "Compressor", "AirTank", "Manifold", "SolenoidValve (1)", "SolenoidValve (2)", "Regulator", "AirFilter", "PneumTube_1", "PneumTube_2", "SensorBracket", "PhotoSensor"
